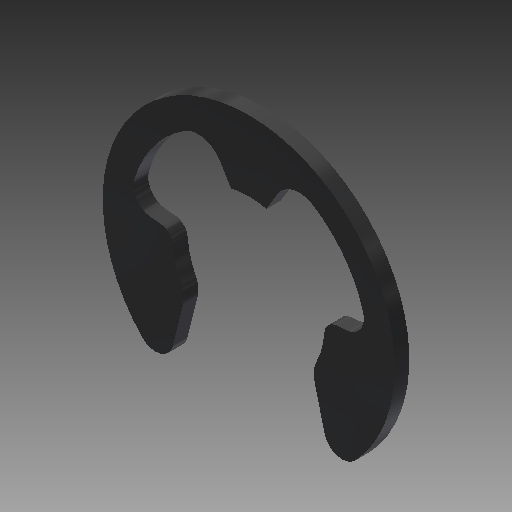
# Autodesk Inventor part: Part19
Saved by Autodesk Inventor 2017.3 (Build 213256000, 256)
## iProperties
Created: 2012-04-08
Part Number: Part19
Material: Steel
Document SubType Name: Modeling
Designer: jhanson2
Density: 7.85 g/cm^3
Appearance: Dark Gray
Mass: 0.328166 g
Surface Area: 1.66776 cm^2
Volume: 0.0418046 cm^3
Author: jhanson2
Autodesk Inventor part; units mm, degrees
ref_plane "YZ Plane" through (0, 0, 0) normal (1, 0, 0) x (0, 1, 0)
ref_plane "XZ Plane" through (0, 0, 0) normal (0, 1, 0) x (-1, 0, 0)
ref_plane "XY Plane" through (0, 0, 0) normal (0, 0, 1) x (1, 0, 0)
sketch "Sketch1" plane through (0, 0, 0) normal (0, 0, 1) x (1, 0, 0)
  arc A0 (5.0089, -4.6844) -> (-5.0089, -4.6844) centre (0, 0) ccw
  line L0 (0, 0) -> (0, 3.3219)
  line L1 (0, 0) -> (0, -6.858)
  line L2 (4.1269, 0.3611) -> (4.5966, 0.4021)
  line L3 (-4.1269, 0.3611) -> (-4.5966, 0.4021)
  line L4 (-3.0829, -2.3997) -> (-3.5588, -4.3082)
  line L5 (3.0829, -2.3997) -> (3.5588, -4.3082)
  arc A1 (0.8337, 3.4569) -> (-0.8337, 3.4569) centre (0, 0) ccw
  arc A2 (-3.5485, -0.2304) -> (-3.1723, -1.6067) centre (0, 0) ccw
  arc A3 (3.1723, -1.6067) -> (3.5485, -0.2304) centre (0, 0) ccw
  arc A4 (3.5588, -4.3082) -> (5.0089, -4.6844) centre (4.3861, -4.102) ccw
  arc A5 (-5.0089, -4.6844) -> (-3.5588, -4.3082) centre (-4.3861, -4.102) ccw
  arc A6 (4.1269, 0.3611) -> (3.5485, -0.2304) centre (4.1822, -0.2715) ccw
  arc A7 (3.1723, -1.6067) -> (3.0829, -2.3997) centre (4.192, -2.1232) ccw
  arc A8 (-3.5485, -0.2304) -> (-4.1269, 0.3611) centre (-4.1822, -0.2715) ccw
  arc A9 (-3.0829, -2.3997) -> (-3.1723, -1.6067) centre (-4.192, -2.1232) ccw
  arc A10 (4.5966, 0.4021) -> (5.3741, 1.5314) centre (4.5191, 1.2878) ccw
  arc A11 (3.0157, 4.7044) -> (1.3489, 4.3144) centre (2.3718, 3.6998) ccw
  arc A12 (-5.3741, 1.5314) -> (-4.5966, 0.4021) centre (-4.5191, 1.2878) ccw
  arc A13 (-1.3489, 4.3144) -> (-3.0157, 4.7044) centre (-2.3718, 3.6998) ccw
  line L6 (-0.8337, 3.4569) -> (-1.3489, 4.3144)
  line L7 (0.8337, 3.4569) -> (1.3489, 4.3144)
  arc A14 (5.3741, 1.5314) -> (3.0157, 4.7044) centre (0, 0) ccw
  arc A15 (-3.0157, 4.7044) -> (-5.3741, 1.5314) centre (0, 0) ccw
  point P0 (5.5667, 0.487)
  point P1 (-5.5667, 0.487)
  point P2 (-3.7479, -5.1854)
  point P3 (2.9716, -1.9532)
  point P4 (3.7479, -5.1854)
  point P5 (1.4868, 5.1225)
  point P6 (0, 2.4453)
  point P7 (-1.4868, 5.1225)
  point P8 (0, 2.4453)
  point P9 (-2.9716, -1.9532)
  point P10 (-0.8419, 3.4705)
  point P11 (-2.3046, 5.9049)
  point P12 (0.8419, 3.4705)
  point P13 (2.3046, 5.9049)
  dimension "d0" = 13.716
  dimension "d2" = 95
  dimension "d3" = 14
  dimension "d4" = 3.556
  dimension "d5" = 0.8527
  dimension "d6" = 3.556
  dimension "d7" = 14
  dimension "d8" = 1.27
  dimension "d9" = 1.27
  dimension "d10" = 1.778
  dimension "d11" = 31
  dimension "d12" = 2.286
  constraints: 32 point on circle, 16 centre point, 16 end point, 16 tangent, 7 symmetric about line, 3 coincident, 3 equal radius, 3 point on line, 1 collinear
  measures "d0" diameter of A0
  measures "d2" angle of L1 L2
  measures "d3" angle of L1 L5
  measures "d4" radius of A1
  measures "d5" radius of A4
  measures "d6" radius of A2
  measures "d7" angle of L1 L4
  measures "d8" diameter of A6
  measures "d9" diameter of A8
  measures "d10" diameter of A10
  measures "d11" angle of L7 L0
  measures "d12" diameter of A7
extrude "Extrusion1" add sketch "Sketch1" along normal blind 0.6858
equation "\"d6\" = d4"
equation "\"d7\" = d3"
equation "\"d9\" = d8"
body "Solid1"
